Autodesk Fusion 360 part; units mm, degrees
(part 2 of 4)
  spline S375 degree 3 poles (7.1269, -2.7048) (6.3878, -3.105) (5.6098, -3.3959) (4.7931, -3.5774) knots 0 0 0 0 1 1 1 1
  spline S376 degree 3 poles (4.7931, -3.5774) (3.8693, -3.6414) (3.3958, -3.2084) (3.3726, -2.2787) knots 0 0 0 0 1 1 1 1
  spline S377 degree 3 poles (3.3726, -2.2787) (3.372, -1.9493) (3.4329, -1.6314) (3.5552, -1.3249) knots 0 0 0 0 1 1 1 1
  spline S378 degree 3 poles (3.5552, -1.3249) (3.871, -0.6919) (4.243, -0.0966) (4.6713, 0.4609) knots 0 0 0 0 1 1 1 1
  spline S379 degree 3 poles (4.6713, 0.4609) (4.606, 0.4941) (4.5384, 0.5211) (4.4684, 0.5421) knots 0 0 0 0 1 1 1 1
  spline S380 degree 3 poles (4.4684, 0.5421) (3.6102, -0.7693) (2.5279, -1.8584) (1.2215, -2.7251) knots 0 0 0 0 1 1 1 1
  spline S381 degree 3 poles (1.2215, -2.7251) (0.6448, -3.0748) (0.0225, -3.271) (-0.6454, -3.3136) knots 0 0 0 0 1 1 1 1
  spline S382 degree 3 poles (-0.6454, -3.3136) (-1.1329, -3.3261) (-1.4711, -3.1097) (-1.6601, -2.6642) knots 0 0 0 0 1 1 1 1
  spline S383 degree 3 poles (-1.6601, -2.6642) (-2.1725, -3.0359) (-2.7407, -3.2862) (-3.3647, -3.4151) knots 0 0 0 0 1 1 1 1
  spline S384 degree 3 poles (-3.3647, -3.4151) (-4.1602, -3.5477) (-4.8163, -3.3109) (-5.3331, -2.7048) knots 0 0 0 0 1 1 1 1
  spline S385 degree 3 poles (-5.3331, -2.7048) (-5.4007, -2.5695) (-5.4684, -2.4342) (-5.536, -2.299) knots 0 0 0 0 1 1 1 1
  spline S386 degree 3 poles (-5.536, -2.299) (-6.3793, -2.8663) (-7.2655, -3.3668) (-8.1944, -3.8006) knots 0 0 0 0 1 1 1 1
  spline S387 degree 3 poles (-8.1944, -3.8006) (-8.9496, -5.1315) (-9.8831, -6.3288) (-10.9948, -7.3925) knots 0 0 0 0 1 1 1 1
  spline S388 degree 3 poles (-10.9948, -7.3925) (-11.4326, -7.767) (-11.9332, -8.024) (-12.4965, -8.1636) knots 0 0 0 0 1 1 1 1
  spline S389 degree 3 poles (-12.4965, -8.1636) (-13.0579, -8.2343) (-13.4434, -8.0111) (-13.6532, -7.4939) knots 0 0 0 0 1 1 1 1
  spline S390 degree 3 poles (-13.6532, -7.4939) (-13.7714, -6.9994) (-13.7173, -6.5258) (-13.4908, -6.0734) knots 0 0 0 0 1 1 1 1
  spline S391 degree 3 poles (-13.4908, -6.0734) (-13.178, -5.5846) (-12.7924, -5.1584) (-12.3341, -4.795) knots 0 0 0 0 1 1 1 1
  spline S392 degree 3 poles (-12.3341, -4.795) (-11.6938, -4.29) (-11.0309, -3.8165) (-10.3454, -3.3745) knots 0 0 0 0 1 1 1 1
  spline S393 degree 3 poles (-10.3454, -3.3745) (-11.0952, -3.3991) (-11.6363, -3.0812) (-11.9689, -2.4207) knots 0 0 0 0 1 1 1 1
  spline S394 degree 3 poles (-11.9689, -2.4207) (-12.5057, -2.7974) (-13.0874, -3.0882) (-13.714, -3.2933) knots 0 0 0 0 1 1 1 1
  spline S395 degree 3 poles (-13.714, -3.2933) (-14.134, -3.37) (-14.5534, -3.37) (-14.9722, -3.2933) knots 0 0 0 0 1 1 1 1
  spline S396 degree 3 poles (-14.9722, -3.2933) (-15.2294, -3.1914) (-15.4458, -3.0358) (-15.6216, -2.8266) knots 0 0 0 0 1 1 1 1
  spline S397 degree 3 poles (-15.6216, -2.8266) (-16.2636, -3.2954) (-16.9806, -3.5051) (-17.7726, -3.4556) knots 0 0 0 0 1 1 1 1
  spline S398 degree 3 poles (-17.7726, -3.4556) (-18.8257, -3.1842) (-19.3196, -2.501) (-19.254, -1.4061) knots 0 0 0 0 1 1 1 1
  spline S399 degree 3 poles (-19.254, -1.4061) (-20.4254, -3.0432) (-22.0015, -3.6587) (-23.9822, -3.2527) knots 0 0 0 0 1 1 1 1
  spline S400 degree 3 poles (-23.9822, -3.2527) (-25.2943, -2.7924) (-25.9098, -1.8656) (-25.8289, -0.4726) knots 0 0 0 0 1 1 1 1
  spline S401 degree 3 poles (-25.8289, -0.4726) (-26.3281, -1.486) (-26.9843, -2.3856) (-27.7973, -3.1715) knots 0 0 0 0 1 1 1 1
  spline S402 degree 3 poles (-27.7973, -3.1715) (-28.5299, -3.7639) (-29.3551, -3.9533) (-30.273, -3.7397) knots 0 0 0 0 1 1 1 1
  spline S403 degree 3 poles (-30.273, -3.7397) (-30.803, -3.533) (-31.1886, -3.1745) (-31.4297, -2.6642) knots 0 0 0 0 1 1 1 1
  spline S404 degree 3 poles (-31.4297, -2.6642) (-31.4909, -2.3828) (-31.5044, -2.0987) (-31.4703, -1.8119) knots 0 0 0 0 1 1 1 1
  spline S405 degree 3 poles (-31.4703, -1.8119) (-31.2781, -1.361) (-30.9602, -1.246) (-30.5166, -1.4669) knots 0 0 0 0 1 1 1 1
  spline S406 degree 3 poles (-30.5166, -1.4669) (-30.4692, -1.5143) (-30.4219, -1.5616) (-30.3745, -1.609) knots 0 0 0 0 1 1 1 1
  spline S407 degree 3 poles (-30.3745, -1.609) (-30.3009, -1.7897) (-30.2197, -1.9656) (-30.131, -2.1366) knots 0 0 0 0 1 1 1 1
  spline S408 degree 3 poles (-30.131, -2.1366) (-29.5892, -2.3943) (-29.0819, -2.3335) (-28.609, -1.954) knots 0 0 0 0 1 1 1 1
  spline S409 degree 3 poles (-28.609, -1.954) (-28.0451, -1.3869) (-27.5648, -0.7579) (-27.1682, -0.0667) knots 0 0 0 0 1 1 1 1
  spline S410 degree 3 poles (-27.1682, -0.0667) (-26.4362, 1.3739) (-25.6313, 2.7674) (-24.7534, 4.1136) knots 0 0 0 0 1 1 1 1
  spline S411 degree 3 poles (-24.7534, 4.1136) (-25.9222, 4.7434) (-26.3213, 5.704) (-25.9507, 6.9952) knots 0 0 0 0 1 1 1 1
  spline S412 degree 3 poles (-25.9507, 6.9952) (-25.459, 8.0956) (-24.6134, 8.7111) (-23.414, 8.8418) knots 0 0 0 0 1 1 1 1
  spline S413 degree 3 poles (-23.414, 8.8418) (-22.6035, 8.8984) (-21.8189, 8.7834) (-21.0601, 8.4969) knots 0 0 0 0 1 1 1 1
  spline S414 degree 3 poles (-21.0601, 8.4969) (-20.2808, 9.0289) (-19.4285, 9.3671) (-18.5032, 9.5115) knots 0 0 0 0 1 1 1 1
  spline S415 degree 3 poles (-23.1299, 7.1575) (-23.7547, 7.0989) (-24.2485, 6.8148) (-24.6113, 6.3052) knots 0 0 0 0 1 1 1 1
  spline S416 degree 3 poles (-24.6113, 6.3052) (-24.6371, 6.2186) (-24.6235, 6.1374) (-24.5707, 6.0617) knots 0 0 0 0 1 1 1 1
  spline S417 degree 3 poles (-24.5707, 6.0617) (-24.4029, 5.8532) (-24.1932, 5.7247) (-23.9417, 5.6762) knots 0 0 0 0 1 1 1 1
  spline S418 degree 3 poles (-23.9417, 5.6762) (-23.5939, 6.1864) (-23.2151, 6.6734) (-22.8053, 7.1372) knots 0 0 0 0 1 1 1 1
  spline S419 degree 3 poles (-22.8053, 7.1372) (-22.9127, 7.1574) (-23.0209, 7.1642) (-23.1299, 7.1575) knots 0 0 0 0 1 1 1 1
  spline S420 degree 3 poles (-19.7207, 5.5341) (-19.7709, 5.4204) (-19.8317, 5.3122) (-19.9034, 5.2094) knots 0 0 0 0 1 1 1 1
  spline S421 degree 3 poles (-19.9034, 5.2094) (-20.3499, 4.7732) (-20.8437, 4.4012) (-21.3848, 4.0933) knots 0 0 0 0 1 1 1 1
  spline S422 degree 3 poles (-21.3848, 4.0933) (-21.9574, 3.7979) (-22.5662, 3.6356) (-23.2111, 3.6063) knots 0 0 0 0 1 1 1 1
  spline S423 degree 3 poles (-23.2111, 3.6063) (-23.6736, 2.9136) (-24.12, 2.2102) (-24.5504, 1.4958) knots 0 0 0 0 1 1 1 1
  spline S424 degree 3 poles (-24.5504, 1.4958) (-23.8967, 1.5933) (-23.2474, 1.5527) (-22.6023, 1.3741) knots 0 0 0 0 1 1 1 1
  spline S425 degree 3 poles (-22.6023, 1.3741) (-21.7597, 1.1706) (-21.4688, 0.6498) (-21.7297, -0.1885) knots 0 0 0 0 1 1 1 1
  spline S426 degree 3 poles (-21.7297, -0.1885) (-21.8822, -0.4816) (-22.1257, -0.6439) (-22.4603, -0.6755) knots 0 0 0 0 1 1 1 1
  spline S427 degree 3 poles (-22.4603, -0.6755) (-22.7996, -0.5567) (-23.1446, -0.4552) (-23.4952, -0.3711) knots 0 0 0 0 1 1 1 1
  spline S428 degree 3 poles (-23.4952, -0.3711) (-23.6981, -0.3441) (-23.9011, -0.3441) (-24.104, -0.3711) knots 0 0 0 0 1 1 1 1
  spline S429 degree 3 poles (-24.104, -0.3711) (-24.2834, -0.4288) (-24.3916, -0.5506) (-24.4287, -0.7364) knots 0 0 0 0 1 1 1 1
  spline S430 degree 3 poles (-24.4287, -0.7364) (-24.3891, -0.9653) (-24.2809, -1.1547) (-24.104, -1.3046) knots 0 0 0 0 1 1 1 1
  spline S431 degree 3 poles (-24.104, -1.3046) (-23.5604, -1.6749) (-22.9651, -1.7831) (-22.3182, -1.6293) knots 0 0 0 0 1 1 1 1
  spline S432 degree 3 poles (-22.3182, -1.6293) (-21.5751, -1.43) (-20.9595, -1.0309) (-20.4716, -0.432) knots 0 0 0 0 1 1 1 1
  spline S433 degree 3 poles (-20.4716, -0.432) (-19.3498, 1.1058) (-18.9575, 2.8104) (-19.2946, 4.6818) knots 0 0 0 0 1 1 1 1
  spline S434 degree 3 poles (-19.2946, 4.6818) (-19.3737, 5.0024) (-19.5157, 5.2865) (-19.7207, 5.5341) knots 0 0 0 0 1 1 1 1
  spline S435 degree 3 poles (3.1696, 1.6785) (2.4119, 0.9411) (1.634, 0.2241) (0.836, -0.4726) knots 0 0 0 0 1 1 1 1
  spline S436 degree 3 poles (0.836, -0.4726) (0.6736, -0.7161) (0.5113, -0.9596) (0.3489, -1.2031) knots 0 0 0 0 1 1 1 1
  spline S437 degree 3 poles (0.3489, -1.2031) (0.3091, -1.2542) (0.2956, -1.3083) (0.3083, -1.3655) knots 0 0 0 0 1 1 1 1
  spline S438 degree 3 poles (0.3083, -1.3655) (1.4523, -0.6846) (2.3993, 0.2083) (3.1493, 1.3132) knots 0 0 0 0 1 1 1 1
  spline S439 degree 3 poles (3.1493, 1.3132) (3.2168, 1.4374) (3.2236, 1.5591) (3.1696, 1.6785) knots 0 0 0 0 1 1 1 1
  spline S440 degree 3 poles (10.7999, 0.8667) (10.5828, 0.7924) (10.3665, 0.7045) (10.1506, 0.6029) knots 0 0 0 0 1 1 1 1
  spline S441 degree 3 poles (10.1506, 0.6029) (10.5418, 0.5621) (10.9071, 0.6432) (11.2464, 0.8464) knots 0 0 0 0 1 1 1 1
  spline S442 degree 3 poles (11.2464, 0.8464) (11.0982, 0.8667) (10.9493, 0.8734) (10.7999, 0.8667) knots 0 0 0 0 1 1 1 1
  spline S443 degree 3 poles (-1.1325, 0.6232) (-2.2555, 0.3285) (-3.2092, -0.2533) (-3.9938, -1.122) knots 0 0 0 0 1 1 1 1
  spline S444 degree 3 poles (-3.9938, -1.122) (-4.1157, -1.269) (-4.1969, -1.4313) (-4.2373, -1.609) knots 0 0 0 0 1 1 1 1
  spline S445 degree 3 poles (-4.2373, -1.609) (-4.1708, -1.7027) (-4.0829, -1.7636) (-3.9735, -1.7916) knots 0 0 0 0 1 1 1 1
  spline S446 degree 3 poles (-3.9735, -1.7916) (-3.69, -1.836) (-3.4194, -1.7954) (-3.1617, -1.6699) knots 0 0 0 0 1 1 1 1
  spline S447 degree 3 poles (-3.1617, -1.6699) (-2.1944, -1.1222) (-1.3624, -0.4119) (-0.6657, 0.4609) knots 0 0 0 0 1 1 1 1
  spline S448 degree 3 poles (-0.6657, 0.4609) (-0.6205, 0.512) (-0.6138, 0.5594) (-0.6454, 0.6029) knots 0 0 0 0 1 1 1 1
  spline S449 degree 3 poles (-0.6454, 0.6029) (-0.8072, 0.6232) (-0.9695, 0.63) (-1.1325, 0.6232) knots 0 0 0 0 1 1 1 1
  spline S450 degree 3 poles (-14.8099, 0.5826) (-16.001, 0.2541) (-16.9818, -0.3953) (-17.7523, -1.3655) knots 0 0 0 0 1 1 1 1
  spline S451 degree 3 poles (-17.7523, -1.3655) (-17.916, -1.5781) (-17.8686, -1.7202) (-17.6103, -1.7916) knots 0 0 0 0 1 1 1 1
  spline S452 degree 3 poles (-17.6103, -1.7916) (-17.4615, -1.8187) (-17.3127, -1.8187) (-17.1638, -1.7916) knots 0 0 0 0 1 1 1 1
  spline S453 degree 3 poles (-17.1638, -1.7916) (-16.7697, -1.6554) (-16.4044, -1.4661) (-16.068, -1.2234) knots 0 0 0 0 1 1 1 1
  spline S454 degree 3 poles (-16.068, -1.2234) (-15.3561, -0.7146) (-14.7067, -0.1328) (-14.1199, 0.5218) knots 0 0 0 0 1 1 1 1
  spline S455 degree 3 poles (-14.1199, 0.5218) (-14.3424, 0.5806) (-14.5724, 0.6009) (-14.8099, 0.5826) knots 0 0 0 0 1 1 1 1
  spline S456 degree 3 poles (16.8878, 0.5826) (16.6881, 0.5291) (16.4852, 0.4682) (16.279, 0.4) knots 0 0 0 0 1 1 1 1
  spline S457 degree 3 poles (16.279, 0.4) (15.2944, -0.0031) (14.4896, -0.6321) (13.8642, -1.4872) knots 0 0 0 0 1 1 1 1
  spline S458 degree 3 poles (13.8642, -1.4872) (13.8341, -1.566) (13.8406, -1.6404) (13.8844, -1.7105) knots 0 0 0 0 1 1 1 1
  spline S459 degree 3 poles (13.8844, -1.7105) (14.1799, -1.8416) (14.4774, -1.8416) (14.7773, -1.7105) knots 0 0 0 0 1 1 1 1
  spline S460 degree 3 poles (14.7773, -1.7105) (15.1357, -1.5382) (15.4738, -1.3352) (15.792, -1.1017) knots 0 0 0 0 1 1 1 1
  spline S461 degree 3 poles (15.792, -1.1017) (16.4174, -0.6385) (16.9925, -0.1177) (17.5169, 0.4609) knots 0 0 0 0 1 1 1 1
  spline S462 degree 3 poles (17.5169, 0.4609) (17.5364, 0.4994) (17.5433, 0.5399) (17.5372, 0.5826) knots 0 0 0 0 1 1 1 1
  spline S463 degree 3 poles (17.5372, 0.5826) (17.3208, 0.5826) (17.1041, 0.5826) (16.8878, 0.5826) knots 0 0 0 0 1 1 1 1
  spline S464 degree 3 poles (11.0029, -1.2031) (10.1522, -1.325) (9.3271, -1.2303) (8.5271, -0.919) knots 0 0 0 0 1 1 1 1
  spline S465 degree 3 poles (8.5271, -0.919) (8.4602, -0.9709) (8.4127, -1.0386) (8.3851, -1.122) knots 0 0 0 0 1 1 1 1
  spline S466 degree 3 poles (8.3851, -1.122) (8.3376, -1.264) (8.2901, -1.4061) (8.243, -1.5481) knots 0 0 0 0 1 1 1 1
  spline S467 degree 3 poles (8.243, -1.5481) (8.2532, -1.5993) (8.2804, -1.6399) (8.3242, -1.6699) knots 0 0 0 0 1 1 1 1
  spline S468 degree 3 poles (8.3242, -1.6699) (9.2719, -1.8362) (10.1648, -1.6806) (11.0029, -1.2031) knots 0 0 0 0 1 1 1 1
  spline S469 degree 3 poles (-18.5032, 9.3492) (-17.6562, 9.4316) (-16.858, 9.276) (-16.1086, 8.8824) knots 0 0 0 0 1 1 1 1
  spline S470 degree 3 poles (-16.1086, 8.8824) (-15.7821, 8.6642) (-15.5454, 8.3733) (-15.3984, 8.0098) knots 0 0 0 0 1 1 1 1
  spline S471 degree 3 poles (-15.3984, 8.0098) (-15.3446, 7.5901) (-15.5273, 7.394) (-15.9463, 7.4213) knots 0 0 0 0 1 1 1 1
  spline S472 degree 3 poles (-15.9463, 7.4213) (-16.0104, 7.45) (-16.0713, 7.4838) (-16.1289, 7.5228) knots 0 0 0 0 1 1 1 1
  spline S473 degree 3 poles (-16.1289, 7.5228) (-16.3363, 8.0225) (-16.7083, 8.3133) (-17.245, 8.3954) knots 0 0 0 0 1 1 1 1
  spline S474 degree 3 poles (-17.245, 8.3954) (-18.2437, 8.5762) (-19.1772, 8.4071) (-20.0454, 7.8881) knots 0 0 0 0 1 1 1 1
  spline S475 degree 3 poles (-20.0454, 7.8881) (-18.6024, 6.8964) (-17.8854, 5.5164) (-17.8944, 3.7483) knots 0 0 0 0 1 1 1 1
  spline S476 degree 3 poles (-17.8944, 3.7483) (-17.9234, 1.9636) (-18.4442, 0.3401) (-19.4569, -1.122) knots 0 0 0 0 1 1 1 1
  spline S477 degree 3 poles (-19.4569, -1.122) (-20.0686, -1.91) (-20.8465, -2.4579) (-21.7906, -2.7657) knots 0 0 0 0 1 1 1 1
  spline S478 degree 3 poles (-21.7906, -2.7657) (-22.926, -3.1064) (-23.9677, -2.9305) (-24.9157, -2.2381) knots 0 0 0 0 1 1 1 1
  spline S479 degree 3 poles (-24.9157, -2.2381) (-25.5232, -1.656) (-25.7599, -0.9457) (-25.626, -0.1073) knots 0 0 0 0 1 1 1 1
  spline S480 degree 3 poles (-25.626, -0.1073) (-25.4125, 0.6474) (-24.9186, 1.087) (-24.1446, 1.2117) knots 0 0 0 0 1 1 1 1
  spline S481 degree 3 poles (-24.1446, 1.2117) (-23.6207, 1.2236) (-23.1066, 1.156) (-22.6023, 1.0088) knots 0 0 0 0 1 1 1 1
  spline S482 degree 3 poles (-22.6023, 1.0088) (-22.3358, 0.9581) (-22.1397, 0.816) (-22.0138, 0.5826) knots 0 0 0 0 1 1 1 1
  spline S483 degree 3 poles (-22.0138, 0.5826) (-21.9865, 0.1636) (-22.1826, -0.019) (-22.6023, 0.0347) knots 0 0 0 0 1 1 1 1
  spline S484 degree 3 poles (-22.6023, 0.0347) (-23.1335, 0.2942) (-23.6882, 0.3754) (-24.2664, 0.2782) knots 0 0 0 0 1 1 1 1
  spline S485 degree 3 poles (-24.2664, 0.2782) (-24.6176, 0.1035) (-24.7799, -0.1806) (-24.7534, -0.5741) knots 0 0 0 0 1 1 1 1
  spline S486 degree 3 poles (-24.7534, -0.5741) (-24.7601, -1.0409) (-24.5707, -1.4061) (-24.1852, -1.6699) knots 0 0 0 0 1 1 1 1
  spline S487 degree 3 poles (-24.1852, -1.6699) (-23.6603, -1.9874) (-23.0921, -2.0957) (-22.4806, -1.9946) knots 0 0 0 0 1 1 1 1
  spline S488 degree 3 poles (-22.4806, -1.9946) (-21.5608, -1.8425) (-20.81, -1.4028) (-20.2281, -0.6755) knots 0 0 0 0 1 1 1 1
  spline S489 degree 3 poles (-20.2281, -0.6755) (-19.4037, 0.4439) (-18.9302, 1.702) (-18.8076, 3.099) knots 0 0 0 0 1 1 1 1
  spline S490 degree 3 poles (-18.8076, 3.099) (-18.6631, 4.1951) (-18.8796, 5.2098) (-19.4569, 6.1429) knots 0 0 0 0 1 1 1 1
  spline S491 degree 3 poles (-19.4569, 6.1429) (-19.8338, 6.6553) (-20.3072, 7.0476) (-20.8774, 7.3199) knots 0 0 0 0 1 1 1 1
  spline S492 degree 3 poles (-20.8774, 7.3199) (-21.5825, 6.7128) (-22.198, 6.0296) (-22.7241, 5.2703) knots 0 0 0 0 1 1 1 1
  spline S493 degree 3 poles (-22.7241, 5.2703) (-22.397, 5.3207) (-22.0859, 5.429) (-21.7906, 5.595) knots 0 0 0 0 1 1 1 1
  spline S494 degree 3 poles (-21.7906, 5.595) (-21.4151, 5.8621) (-21.0633, 6.1598) (-20.7354, 6.4879) knots 0 0 0 0 1 1 1 1
  spline S495 degree 3 poles (-20.7354, 6.4879) (-20.4696, 6.6428) (-20.2464, 6.5955) (-20.0657, 6.3458) knots 0 0 0 0 1 1 1 1
  spline S496 degree 3 poles (-20.0657, 6.3458) (-20.0235, 6.1453) (-20.0505, 5.9559) (-20.1469, 5.7776) knots 0 0 0 0 1 1 1 1
  spline S497 degree 3 poles (-20.1469, 5.7776) (-21.0651, 4.845) (-22.1745, 4.3174) (-23.4749, 4.1948) knots 0 0 0 0 1 1 1 1
  spline S498 degree 3 poles (-23.4749, 4.1948) (-23.8673, 3.5725) (-24.2596, 2.9501) (-24.6519, 2.3278) knots 0 0 0 0 1 1 1 1
  spline S499 degree 3 poles (-24.6519, 2.3278) (-25.318, 1.1172) (-25.9945, -0.0868) (-26.6812, -1.2843) knots 0 0 0 0 1 1 1 1
  spline S500 degree 3 poles (-26.6812, -1.2843) (-26.996, -1.7575) (-27.3545, -2.1972) (-27.7567, -2.6033) knots 0 0 0 0 1 1 1 1
  spline S501 degree 3 poles (-27.7567, -2.6033) (-28.3894, -3.1795) (-29.1335, -3.423) (-29.9889, -3.3339) knots 0 0 0 0 1 1 1 1
  spline S502 degree 3 poles (-29.9889, -3.3339) (-30.5331, -3.1815) (-30.9457, -2.8636) (-31.2268, -2.3801) knots 0 0 0 0 1 1 1 1
  spline S503 degree 3 poles (-31.2268, -2.3801) (-31.3301, -2.1673) (-31.3437, -1.9508) (-31.2674, -1.7308) knots 0 0 0 0 1 1 1 1
  spline S504 degree 3 poles (-31.2674, -1.7308) (-31.061, -1.5028) (-30.8243, -1.469) (-30.5571, -1.6293) knots 0 0 0 0 1 1 1 1
  spline S505 degree 3 poles (-30.5571, -1.6293) (-30.4671, -1.791) (-30.3927, -1.9601) (-30.3339, -2.1366) knots 0 0 0 0 1 1 1 1
  spline S506 degree 3 poles (-30.3339, -2.1366) (-30.0544, -2.4455) (-29.7094, -2.547) (-29.299, -2.441) knots 0 0 0 0 1 1 1 1
  spline S507 degree 3 poles (-29.299, -2.441) (-28.8702, -2.3503) (-28.5117, -2.1406) (-28.2235, -1.8119) knots 0 0 0 0 1 1 1 1
  spline S508 degree 3 poles (-28.2235, -1.8119) (-27.8963, -1.4415) (-27.5986, -1.0491) (-27.3306, -0.6349) knots 0 0 0 0 1 1 1 1
  spline S509 degree 3 poles (-27.3306, -0.6349) (-26.7386, 0.4002) (-26.1568, 1.4419) (-25.5854, 2.4902) knots 0 0 0 0 1 1 1 1
  spline S510 degree 3 poles (-25.5854, 2.4902) (-25.1829, 3.1464) (-24.7703, 3.7958) (-24.3475, 4.4383) knots 0 0 0 0 1 1 1 1
  spline S511 degree 3 poles (-24.3475, 4.4383) (-25.5575, 4.8706) (-26.0378, 5.7093) (-25.7883, 6.9546) knots 0 0 0 0 1 1 1 1
  spline S512 degree 3 poles (-25.7883, 6.9546) (-25.3369, 7.9894) (-24.5455, 8.5644) (-23.414, 8.6795) knots 0 0 0 0 1 1 1 1
  spline S513 degree 3 poles (-23.414, 8.6795) (-22.5987, 8.7342) (-21.8073, 8.6191) (-21.0398, 8.3345) knots 0 0 0 0 1 1 1 1
  spline S514 degree 3 poles (-21.0398, 8.3345) (-20.261, 8.8494) (-19.4155, 9.1876) (-18.5032, 9.3492) knots 0 0 0 0 1 1 1 1
  spline S515 degree 3 poles (-23.1299, 7.1575) (-23.7547, 7.0989) (-24.2485, 6.8148) (-24.6113, 6.3052) knots 0 0 0 0 1 1 1 1
  spline S516 degree 3 poles (-24.6113, 6.3052) (-24.6371, 6.2186) (-24.6235, 6.1374) (-24.5707, 6.0617) knots 0 0 0 0 1 1 1 1
  spline S517 degree 3 poles (-24.5707, 6.0617) (-24.4029, 5.8532) (-24.1932, 5.7247) (-23.9417, 5.6762) knots 0 0 0 0 1 1 1 1
  spline S518 degree 3 poles (-23.9417, 5.6762) (-23.5939, 6.1864) (-23.2151, 6.6734) (-22.8053, 7.1372) knots 0 0 0 0 1 1 1 1
  spline S519 degree 3 poles (-22.8053, 7.1372) (-22.9127, 7.1574) (-23.0209, 7.1642) (-23.1299, 7.1575) knots 0 0 0 0 1 1 1 1
  spline S520 degree 3 poles (-23.3735, 7.8069) (-23.1026, 7.8136) (-22.832, 7.8069) (-22.5617, 7.7866) knots 0 0 0 0 1 1 1 1
  spline S521 degree 3 poles (-22.5617, 7.7866) (-22.3197, 7.7733) (-22.0897, 7.7192) (-21.8718, 7.6243) knots 0 0 0 0 1 1 1 1
  spline S522 degree 3 poles (-21.8718, 7.6243) (-22.5639, 6.9085) (-23.193, 6.1441) (-23.759, 5.3312) knots 0 0 0 0 1 1 1 1
  spline S523 degree 3 poles (-23.759, 5.3312) (-23.789, 5.2876) (-23.8296, 5.2605) (-23.8808, 5.25) knots 0 0 0 0 1 1 1 1
  spline S524 degree 3 poles (-23.8808, 5.25) (-24.3842, 5.3593) (-24.7495, 5.6434) (-24.9766, 6.1023) knots 0 0 0 0 1 1 1 1
  spline S525 degree 3 poles (-24.9766, 6.1023) (-25.0395, 6.4115) (-24.9854, 6.6956) (-24.8143, 6.9546) knots 0 0 0 0 1 1 1 1
  spline S526 degree 3 poles (-24.8143, 6.9546) (-24.4328, 7.4123) (-23.9525, 7.6964) (-23.3735, 7.8069) knots 0 0 0 0 1 1 1 1
  spline S527 degree 3 poles (-23.1299, 7.1575) (-23.7547, 7.0989) (-24.2485, 6.8148) (-24.6113, 6.3052) knots 0 0 0 0 1 1 1 1
  spline S528 degree 3 poles (-24.6113, 6.3052) (-24.6371, 6.2186) (-24.6235, 6.1374) (-24.5707, 6.0617) knots 0 0 0 0 1 1 1 1
  spline S529 degree 3 poles (-24.5707, 6.0617) (-24.4029, 5.8532) (-24.1932, 5.7247) (-23.9417, 5.6762) knots 0 0 0 0 1 1 1 1
  spline S530 degree 3 poles (-23.9417, 5.6762) (-23.5939, 6.1864) (-23.2151, 6.6734) (-22.8053, 7.1372) knots 0 0 0 0 1 1 1 1
  spline S531 degree 3 poles (-22.8053, 7.1372) (-22.9127, 7.1574) (-23.0209, 7.1642) (-23.1299, 7.1575) knots 0 0 0 0 1 1 1 1
  spline S532 degree 3 poles (-23.3735, 7.3199) (-23.0594, 7.3343) (-22.7482, 7.314) (-22.44, 7.259) knots 0 0 0 0 1 1 1 1
  spline S533 degree 3 poles (-22.44, 7.259) (-22.9598, 6.6988) (-23.4333, 6.1036) (-23.8605, 5.4732) knots 0 0 0 0 1 1 1 1
  spline S534 degree 3 poles (-23.8605, 5.4732) (-24.2998, 5.5197) (-24.6177, 5.743) (-24.8143, 6.1429) knots 0 0 0 0 1 1 1 1
  spline S535 degree 3 poles (-24.8143, 6.1429) (-24.7735, 6.4332) (-24.6314, 6.67) (-24.3881, 6.8531) knots 0 0 0 0 1 1 1 1
  spline S536 degree 3 poles (-24.3881, 6.8531) (-24.0772, 7.0759) (-23.739, 7.2315) (-23.3735, 7.3199) knots 0 0 0 0 1 1 1 1
  spline S537 degree 3 poles (-23.1299, 7.1575) (-23.7547, 7.0989) (-24.2485, 6.8148) (-24.6113, 6.3052) knots 0 0 0 0 1 1 1 1
  spline S538 degree 3 poles (-24.6113, 6.3052) (-24.6371, 6.2186) (-24.6235, 6.1374) (-24.5707, 6.0617) knots 0 0 0 0 1 1 1 1
  spline S539 degree 3 poles (-24.5707, 6.0617) (-24.4029, 5.8532) (-24.1932, 5.7247) (-23.9417, 5.6762) knots 0 0 0 0 1 1 1 1
  spline S540 degree 3 poles (-23.9417, 5.6762) (-23.5939, 6.1864) (-23.2151, 6.6734) (-22.8053, 7.1372) knots 0 0 0 0 1 1 1 1
  spline S541 degree 3 poles (-22.8053, 7.1372) (-22.9127, 7.1574) (-23.0209, 7.1642) (-23.1299, 7.1575) knots 0 0 0 0 1 1 1 1
  spline S542 degree 3 poles (-20.8977, 6.7923) (-20.8197, 6.7803) (-20.752, 6.7465) (-20.6948, 6.6908) knots 0 0 0 0 1 1 1 1
  spline S543 degree 3 poles (-20.6948, 6.6908) (-21.0044, 6.4489) (-21.302, 6.1919) (-21.5877, 5.9197) knots 0 0 0 0 1 1 1 1
  spline S544 degree 3 poles (-21.5877, 5.9197) (-21.6905, 5.8412) (-21.7988, 5.787) (-21.9124, 5.7573) knots 0 0 0 0 1 1 1 1
  spline S545 degree 3 poles (-21.9124, 5.7573) (-21.5931, 6.1239) (-21.2549, 6.4689) (-20.8977, 6.7923) knots 0 0 0 0 1 1 1 1
  spline S546 degree 3 poles (-19.8831, 6.0211) (-19.567, 5.7152) (-19.3302, 5.3499) (-19.1728, 4.9253) knots 0 0 0 0 1 1 1 1
  spline S547 degree 3 poles (-19.1728, 4.9253) (-18.7456, 2.9677) (-19.1109, 1.1684) (-20.2687, -0.4726) knots 0 0 0 0 1 1 1 1
  spline S548 degree 3 poles (-20.2687, -0.4726) (-21.0585, -1.5163) (-22.107, -1.9695) (-23.414, -1.8322) knots 0 0 0 0 1 1 1 1
  spline S549 degree 3 poles (-23.414, -1.8322) (-23.8998, -1.7247) (-24.2718, -1.4609) (-24.5302, -1.0408) knots 0 0 0 0 1 1 1 1
  spline S550 degree 3 poles (-24.5302, -1.0408) (-24.6707, -0.4829) (-24.4542, -0.1853) (-23.8808, -0.1479) knots 0 0 0 0 1 1 1 1
  spline S551 degree 3 poles (-23.8808, -0.1479) (-23.4481, -0.1698) (-23.0355, -0.2713) (-22.6429, -0.4523) knots 0 0 0 0 1 1 1 1
  spline S552 degree 3 poles (-22.6429, -0.4523) (-22.1845, -0.5147) (-21.9139, -0.3185) (-21.8312, 0.1362) knots 0 0 0 0 1 1 1 1
  spline S553 degree 3 poles (-21.8312, 0.1362) (-21.758, 0.5319) (-21.8933, 0.8363) (-22.2371, 1.0494) knots 0 0 0 0 1 1 1 1
  spline S554 degree 3 poles (-22.2371, 1.0494) (-22.9866, 1.3584) (-23.7578, 1.4395) (-24.5504, 1.2929) knots 0 0 0 0 1 1 1 1
  spline S555 degree 3 poles (-24.5504, 1.2929) (-24.6825, 1.2512) (-24.8043, 1.1903) (-24.9157, 1.1103) knots 0 0 0 0 1 1 1 1
  spline S556 degree 3 poles (-24.9157, 1.1103) (-24.9572, 1.1306) (-24.9639, 1.1577) (-24.936, 1.1914) knots 0 0 0 0 1 1 1 1
  spline S557 degree 3 poles (-24.936, 1.1914) (-24.4258, 2.0734) (-23.8914, 2.9392) (-23.3329, 3.7889) knots 0 0 0 0 1 1 1 1
  spline S558 degree 3 poles (-23.3329, 3.7889) (-21.9954, 3.8793) (-20.8793, 4.4205) (-19.9846, 5.4123) knots 0 0 0 0 1 1 1 1
  spline S559 degree 3 poles (-19.9846, 5.4123) (-19.8975, 5.6055) (-19.8637, 5.8084) (-19.8831, 6.0211) knots 0 0 0 0 1 1 1 1
  spline S560 degree 3 poles (-19.7207, 5.5341) (-19.7709, 5.4204) (-19.8317, 5.3122) (-19.9034, 5.2094) knots 0 0 0 0 1 1 1 1
  spline S561 degree 3 poles (-19.9034, 5.2094) (-20.3499, 4.7732) (-20.8437, 4.4012) (-21.3848, 4.0933) knots 0 0 0 0 1 1 1 1
  spline S562 degree 3 poles (-21.3848, 4.0933) (-21.9574, 3.7979) (-22.5662, 3.6356) (-23.2111, 3.6063) knots 0 0 0 0 1 1 1 1
  spline S563 degree 3 poles (-23.2111, 3.6063) (-23.6736, 2.9136) (-24.12, 2.2102) (-24.5504, 1.4958) knots 0 0 0 0 1 1 1 1
  spline S564 degree 3 poles (-24.5504, 1.4958) (-23.8967, 1.5933) (-23.2474, 1.5527) (-22.6023, 1.3741) knots 0 0 0 0 1 1 1 1
  spline S565 degree 3 poles (-22.6023, 1.3741) (-21.7597, 1.1706) (-21.4688, 0.6498) (-21.7297, -0.1885) knots 0 0 0 0 1 1 1 1
  spline S566 degree 3 poles (-21.7297, -0.1885) (-21.8822, -0.4816) (-22.1257, -0.6439) (-22.4603, -0.6755) knots 0 0 0 0 1 1 1 1
  spline S567 degree 3 poles (-22.4603, -0.6755) (-22.7996, -0.5567) (-23.1446, -0.4552) (-23.4952, -0.3711) knots 0 0 0 0 1 1 1 1
  spline S568 degree 3 poles (-23.4952, -0.3711) (-23.6981, -0.3441) (-23.9011, -0.3441) (-24.104, -0.3711) knots 0 0 0 0 1 1 1 1
  spline S569 degree 3 poles (-24.104, -0.3711) (-24.2834, -0.4288) (-24.3916, -0.5506) (-24.4287, -0.7364) knots 0 0 0 0 1 1 1 1
  spline S570 degree 3 poles (-24.4287, -0.7364) (-24.3891, -0.9653) (-24.2809, -1.1547) (-24.104, -1.3046) knots 0 0 0 0 1 1 1 1
  spline S571 degree 3 poles (-24.104, -1.3046) (-23.5604, -1.6749) (-22.9651, -1.7831) (-22.3182, -1.6293) knots 0 0 0 0 1 1 1 1
  spline S572 degree 3 poles (-22.3182, -1.6293) (-21.5751, -1.43) (-20.9595, -1.0309) (-20.4716, -0.432) knots 0 0 0 0 1 1 1 1
  spline S573 degree 3 poles (-20.4716, -0.432) (-19.3498, 1.1058) (-18.9575, 2.8104) (-19.2946, 4.6818) knots 0 0 0 0 1 1 1 1
  spline S574 degree 3 poles (-19.2946, 4.6818) (-19.3737, 5.0024) (-19.5157, 5.2865) (-19.7207, 5.5341) knots 0 0 0 0 1 1 1 1
  spline S575 degree 3 poles (25.6543, 1.1914) (25.6413, 1.0535) (25.6547, 0.9182) (25.6949, 0.7856) knots 0 0 0 0 1 1 1 1
  spline S576 degree 3 poles (25.6949, 0.7856) (25.7197, 0.7906) (25.7331, 0.8041) (25.7355, 0.8262) knots 0 0 0 0 1 1 1 1
  spline S577 degree 3 poles (25.7355, 0.8262) (26.3008, 1.3291) (26.9502, 1.6876) (27.6836, 1.9017) knots 0 0 0 0 1 1 1 1
  spline S578 degree 3 poles (27.6836, 1.9017) (28.2465, 2.043) (28.7133, 1.9009) (29.0838, 1.4755) knots 0 0 0 0 1 1 1 1
  spline S579 degree 3 poles (29.0838, 1.4755) (29.111, 1.4214) (29.1378, 1.3673) (29.165, 1.3132) knots 0 0 0 0 1 1 1 1
  spline S580 degree 3 poles (29.165, 1.3132) (29.2364, 0.8962) (29.1686, 0.5039) (28.9621, 0.1362) knots 0 0 0 0 1 1 1 1
  spline S581 degree 3 poles (28.9621, 0.1362) (28.6325, -0.4008) (28.2538, -0.9013) (27.8257, -1.3655) knots 0 0 0 0 1 1 1 1
  spline S582 degree 3 poles (27.8257, -1.3655) (27.6808, -1.5471) (27.5793, -1.75) (27.5213, -1.9743) knots 0 0 0 0 1 1 1 1
  spline S583 degree 3 poles (27.5213, -1.9743) (28.0615, -1.9769) (28.5619, -1.8349) (29.0229, -1.5481) knots 0 0 0 0 1 1 1 1
  spline S584 degree 3 poles (29.0229, -1.5481) (29.5855, -1.1889) (30.1131, -0.783) (30.6058, -0.3305) knots 0 0 0 0 1 1 1 1
  spline S585 degree 3 poles (30.6058, -0.3305) (31.0843, -0.3189) (31.2397, -0.5421) (31.0725, -1.0002) knots 0 0 0 0 1 1 1 1
  spline S586 degree 3 poles (31.0725, -1.0002) (30.2673, -1.8528) (29.3001, -2.4412) (28.1706, -2.7657) knots 0 0 0 0 1 1 1 1
  spline S587 degree 3 poles (28.1706, -2.7657) (27.8865, -2.7928) (27.6024, -2.7928) (27.3183, -2.7657) knots 0 0 0 0 1 1 1 1
  spline S588 degree 3 poles (27.3183, -2.7657) (26.7538, -2.5485) (26.5712, -2.1494) (26.7704, -1.5684) knots 0 0 0 0 1 1 1 1
  spline S589 degree 3 poles (26.7704, -1.5684) (26.8715, -1.3388) (26.9932, -1.1224) (27.1357, -0.919) knots 0 0 0 0 1 1 1 1
  spline S590 degree 3 poles (27.1357, -0.919) (27.4912, -0.5366) (27.8159, -0.1307) (28.1098, 0.2985) knots 0 0 0 0 1 1 1 1
  spline S591 degree 3 poles (28.1098, 0.2985) (28.2104, 0.4664) (28.2916, 0.6422) (28.3533, 0.8262) knots 0 0 0 0 1 1 1 1
  spline S592 degree 3 poles (28.3533, 0.8262) (28.3841, 0.9182) (28.3772, 1.0062) (28.333, 1.09) knots 0 0 0 0 1 1 1 1
  spline S593 degree 3 poles (28.333, 1.09) (28.1434, 1.117) (27.9543, 1.117) (27.7648, 1.09) knots 0 0 0 0 1 1 1 1
  spline S594 degree 3 poles (27.7648, 1.09) (27.0821, 0.8262) (26.4733, 0.4474) (25.9384, -0.0464) knots 0 0 0 0 1 1 1 1
  spline S595 degree 3 poles (25.9384, -0.0464) (24.9822, -0.9481) (24.1165, -1.9222) (23.3409, -2.9686) knots 0 0 0 0 1 1 1 1
  spline S596 degree 3 poles (23.3409, -2.9686) (23.2687, -2.9668) (23.2009, -2.9398) (23.138, -2.8874) knots 0 0 0 0 1 1 1 1
  spline S597 degree 3 poles (23.138, -2.8874) (22.996, -2.7725) (22.8539, -2.6574) (22.7119, -2.5425) knots 0 0 0 0 1 1 1 1
  spline S598 degree 3 poles (22.7119, -2.5425) (22.6847, -2.5019) (22.6847, -2.4613) (22.7119, -2.4207) knots 0 0 0 0 1 1 1 1
  spline S599 degree 3 poles (22.7119, -2.4207) (23.1599, -1.9049) (23.593, -1.3773) (24.0106, -0.8379) knots 0 0 0 0 1 1 1 1
  spline S600 degree 3 poles (24.0106, -0.8379) (24.3779, -0.3606) (24.6482, 0.167) (24.8223, 0.745) knots 0 0 0 0 1 1 1 1
  spline S601 degree 3 poles (24.8223, 0.745) (24.8613, 0.9102) (24.841, 1.0658) (24.7614, 1.2117) knots 0 0 0 0 1 1 1 1
  spline S602 degree 3 poles (24.7614, 1.2117) (24.4481, 1.2484) (24.1506, 1.1943) (23.8685, 1.0494) knots 0 0 0 0 1 1 1 1
  spline S603 degree 3 poles (23.8685, 1.0494) (23.2687, 0.7596) (22.7005, 0.4214) (22.1639, 0.0347) knots 0 0 0 0 1 1 1 1
  spline S604 degree 3 poles (22.1639, 0.0347) (21.638, -0.3693) (21.1241, -0.7887) (20.6217, -1.2234) knots 0 0 0 0 1 1 1 1
  spline S605 degree 3 poles (20.6217, -1.2234) (20.0032, -1.8691) (19.3607, -2.4846) (18.6939, -3.0701) knots 0 0 0 0 1 1 1 1
  spline S606 degree 3 poles (18.6939, -3.0701) (18.5449, -2.9483) (18.3964, -2.8266) (18.2474, -2.7048) knots 0 0 0 0 1 1 1 1
  spline S607 degree 3 poles (18.2474, -2.7048) (17.7502, -2.8778) (17.2429, -2.9116) (16.7254, -2.8063) knots 0 0 0 0 1 1 1 1
  spline S608 degree 3 poles (16.7254, -2.8063) (16.4641, -2.6936) (16.2676, -2.5109) (16.137, -2.2584) knots 0 0 0 0 1 1 1 1
  spline S609 degree 3 poles (16.137, -2.2584) (15.5955, -2.6689) (14.9868, -2.9124) (14.3106, -2.9889) knots 0 0 0 0 1 1 1 1
  spline S610 degree 3 poles (14.3106, -2.9889) (13.3978, -2.9757) (12.8227, -2.5292) (12.5857, -1.6496) knots 0 0 0 0 1 1 1 1
  spline S611 degree 3 poles (12.5857, -1.6496) (11.7748, -2.1903) (10.8953, -2.5758) (9.9476, -2.8063) knots 0 0 0 0 1 1 1 1
  spline S612 degree 3 poles (9.9476, -2.8063) (9.2974, -2.9375) (8.6477, -2.9375) (7.9995, -2.8063) knots 0 0 0 0 1 1 1 1
  spline S613 degree 3 poles (7.9995, -2.8063) (7.648, -2.6849) (7.3842, -2.4617) (7.2081, -2.1366) knots 0 0 0 0 1 1 1 1
  spline S614 degree 3 poles (7.2081, -2.1366) (6.454, -2.5847) (5.6489, -2.9027) (4.7931, -3.0904) knots 0 0 0 0 1 1 1 1
  spline S615 degree 3 poles (4.7931, -3.0904) (4.0331, -3.1844) (3.6137, -2.8529) (3.5349, -2.096) knots 0 0 0 0 1 1 1 1
  spline S616 degree 3 poles (3.5349, -2.096) (3.5916, -1.662) (3.7337, -1.2562) (3.9611, -0.8785) knots 0 0 0 0 1 1 1 1
  spline S617 degree 3 poles (3.9611, -0.8785) (4.3387, -0.2651) (4.7513, 0.3234) (5.1989, 0.887) knots 0 0 0 0 1 1 1 1
  spline S618 degree 3 poles (5.1989, 0.887) (4.9418, 0.9344) (4.6848, 0.9818) (4.4278, 1.0291) knots 0 0 0 0 1 1 1 1
  spline S619 degree 3 poles (4.4278, 1.0291) (4.2269, 0.8067) (4.0443, 0.5632) (3.8799, 0.2985) knots 0 0 0 0 1 1 1 1
  spline S620 degree 3 poles (3.8799, 0.2985) (3.6364, 0.0009) (3.3929, -0.2967) (3.1493, -0.5943) knots 0 0 0 0 1 1 1 1
  spline S621 degree 3 poles (3.1493, -0.5943) (2.557, -1.2244) (1.9008, -1.7723) (1.1809, -2.2381) knots 0 0 0 0 1 1 1 1
  spline S622 degree 3 poles (1.1809, -2.2381) (0.8389, -2.4226) (0.4872, -2.585) (0.1257, -2.7251) knots 0 0 0 0 1 1 1 1
  spline S623 degree 3 poles (0.1257, -2.7251) (-0.2786, -2.8306) (-0.6845, -2.8441) (-1.0919, -2.7657) knots 0 0 0 0 1 1 1 1
  spline S624 degree 3 poles (-1.0919, -2.7657) (-1.3711, -2.5944) (-1.5132, -2.3441) (-1.518, -2.0149) knots 0 0 0 0 1 1 1 1
  spline S625 degree 3 poles (-1.518, -2.0149) (-2.282, -2.716) (-3.1816, -3.0204) (-4.217, -2.928) knots 0 0 0 0 1 1 1 1
  spline S626 degree 3 poles (-4.217, -2.928) (-4.858, -2.7604) (-5.2707, -2.3613) (-5.4548, -1.7308) knots 0 0 0 0 1 1 1 1
  spline S627 degree 3 poles (-5.4548, -1.7308) (-6.3534, -2.3301) (-7.2936, -2.8645) (-8.2756, -3.3339) knots 0 0 0 0 1 1 1 1
  spline S628 degree 3 poles (-8.2756, -3.3339) (-9.013, -4.613) (-9.9058, -5.7764) (-10.9542, -6.8243) knots 0 0 0 0 1 1 1 1
  spline S629 degree 3 poles (-10.9542, -6.8243) (-11.3533, -7.1958) (-11.8133, -7.4664) (-12.3341, -7.636) knots 0 0 0 0 1 1 1 1
  spline S630 degree 3 poles (-12.3341, -7.636) (-13.1638, -7.7801) (-13.5629, -7.4351) (-13.5314, -6.601) knots 0 0 0 0 1 1 1 1
  spline S631 degree 3 poles (-13.5314, -6.601) (-13.4524, -6.3349) (-13.3307, -6.0914) (-13.1661, -5.8705) knots 0 0 0 0 1 1 1 1
  spline S632 degree 3 poles (-13.1661, -5.8705) (-12.8347, -5.4849) (-12.4762, -5.1264) (-12.0906, -4.795) knots 0 0 0 0 1 1 1 1
  spline S633 degree 3 poles (-12.0906, -4.795) (-11.1036, -4.0387) (-10.0619, -3.3622) (-8.9655, -2.7657) knots 0 0 0 0 1 1 1 1
  spline S634 degree 3 poles (-8.9655, -2.7657) (-8.8753, -2.6594) (-8.8145, -2.5445) (-8.7829, -2.4207) knots 0 0 0 0 1 1 1 1
  spline S635 degree 3 poles (-8.7829, -2.4207) (-9.4149, -2.8072) (-10.0981, -2.9493) (-10.8325, -2.8469) knots 0 0 0 0 1 1 1 1
  spline S636 degree 3 poles (-10.8325, -2.8469) (-11.3953, -2.7169) (-11.7403, -2.3719) (-11.8674, -1.8119) knots 0 0 0 0 1 1 1 1
  spline S637 degree 3 poles (-11.8674, -1.8119) (-12.4436, -2.2658) (-13.0862, -2.5972) (-13.7952, -2.8063) knots 0 0 0 0 1 1 1 1
  spline S638 degree 3 poles (-13.7952, -2.8063) (-14.1315, -2.8653) (-14.4697, -2.8788) (-14.8099, -2.8469) knots 0 0 0 0 1 1 1 1
  spline S639 degree 3 poles (-14.8099, -2.8469) (-15.1554, -2.7719) (-15.4057, -2.5757) (-15.5607, -2.2584) knots 0 0 0 0 1 1 1 1
  spline S640 degree 3 poles (-15.5607, -2.2584) (-16.0968, -2.682) (-16.7056, -2.9255) (-17.3871, -2.9889) knots 0 0 0 0 1 1 1 1
  spline S641 degree 3 poles (-17.3871, -2.9889) (-18.5386, -2.9198) (-19.0932, -2.311) (-19.0511, -1.1626) knots 0 0 0 0 1 1 1 1
  spline S642 degree 3 poles (-19.0511, -1.1626) (-18.9093, -0.6489) (-18.6522, -0.2024) (-18.2799, 0.1768) knots 0 0 0 0 1 1 1 1
  spline S643 degree 3 poles (-18.2799, 0.1768) (-17.4808, 0.9859) (-16.5406, 1.5744) (-15.4592, 1.9423) knots 0 0 0 0 1 1 1 1
  spline S644 degree 3 poles (-15.4592, 1.9423) (-14.7726, 2.1501) (-14.0962, 2.1231) (-13.4299, 1.8611) knots 0 0 0 0 1 1 1 1
  spline S645 degree 3 poles (-13.4299, 1.8611) (-12.9721, 1.5926) (-12.7624, 1.1935) (-12.8009, 0.6638) knots 0 0 0 0 1 1 1 1
  spline S646 degree 3 poles (-12.8009, 0.6638) (-12.6002, 0.8751) (-12.3635, 0.936) (-12.0906, 0.8464) knots 0 0 0 0 1 1 1 1
  spline S647 degree 3 poles (-12.0906, 0.8464) (-11.82, 0.6164) (-11.82, 0.3865) (-12.0906, 0.1565) knots 0 0 0 0 1 1 1 1
  spline S648 degree 3 poles (-12.0906, 0.1565) (-12.9639, -0.3379) (-13.7688, -0.9264) (-14.5055, -1.609) knots 0 0 0 0 1 1 1 1
  spline S649 degree 3 poles (-14.5055, -1.609) (-14.5965, -1.7135) (-14.6709, -1.8285) (-14.7287, -1.954) knots 0 0 0 0 1 1 1 1
  spline S650 degree 3 poles (-14.7287, -1.954) (-14.7123, -1.9923) (-14.6852, -2.0194) (-14.6475, -2.0351) knots 0 0 0 0 1 1 1 1
  spline S651 degree 3 poles (-14.6475, -2.0351) (-14.2054, -2.0739) (-13.786, -1.9927) (-13.3894, -1.7916) knots 0 0 0 0 1 1 1 1
  spline S652 degree 3 poles (-13.3894, -1.7916) (-12.685, -1.4428) (-12.056, -0.9897) (-11.5021, -0.432) knots 0 0 0 0 1 1 1 1
  spline S653 degree 3 poles (-11.5021, -0.432) (-10.8474, 0.7367) (-9.9071, 1.5958) (-8.6814, 2.1452) knots 0 0 0 0 1 1 1 1
  spline S654 degree 3 poles (-8.6814, 2.1452) (-8.1756, 2.2085) (-7.9998, 1.9988) (-8.1538, 1.5161) knots 0 0 0 0 1 1 1 1
  spline S655 degree 3 poles (-8.1538, 1.5161) (-8.8418, 1.2026) (-9.4574, 0.7832) (-10.0004, 0.258) knots 0 0 0 0 1 1 1 1
  spline S656 degree 3 poles (-10.0004, 0.258) (-10.2034, 0.0009) (-10.4063, -0.2561) (-10.6092, -0.5132) knots 0 0 0 0 1 1 1 1
  spline S657 degree 3 poles (-10.6092, -0.5132) (-10.7757, -0.7957) (-10.911, -1.0934) (-11.0151, -1.4061) knots 0 0 0 0 1 1 1 1
  spline S658 degree 3 poles (-11.0151, -1.4061) (-11.1056, -1.7325) (-10.9907, -1.9422) (-10.6701, -2.0351) knots 0 0 0 0 1 1 1 1
  spline S659 degree 3 poles (-10.6701, -2.0351) (-10.3976, -2.064) (-10.127, -2.0505) (-9.8584, -1.9946) knots 0 0 0 0 1 1 1 1
  spline S660 degree 3 poles (-9.8584, -1.9946) (-9.1369, -1.7321) (-8.4808, -1.36) (-7.89, -0.8785) knots 0 0 0 0 1 1 1 1
  spline S661 degree 3 poles (-7.89, -0.8785) (-7.4165, -0.0126) (-6.943, 0.8532) (-6.4695, 1.719) knots 0 0 0 0 1 1 1 1
  spline S662 degree 3 poles (-6.4695, 1.719) (-6.199, 2.0742) (-5.854, 2.1756) (-5.4345, 2.0234) knots 0 0 0 0 1 1 1 1
  spline S663 degree 3 poles (-5.4345, 2.0234) (-5.1615, 1.795) (-5.0735, 1.5041) (-5.1707, 1.1508) knots 0 0 0 0 1 1 1 1
  spline S664 degree 3 poles (-5.1707, 1.1508) (-5.3537, 0.6163) (-5.6378, 0.1428) (-6.023, -0.2697) knots 0 0 0 0 1 1 1 1
  spline S665 degree 3 poles (-6.023, -0.2697) (-6.4045, -0.6782) (-6.8103, -1.057) (-7.2406, -1.4061) knots 0 0 0 0 1 1 1 1
  spline S666 degree 3 poles (-7.2406, -1.4061) (-7.3732, -1.6171) (-7.4815, -1.8336) (-7.5653, -2.0554) knots 0 0 0 0 1 1 1 1
  spline S667 degree 3 poles (-7.5653, -2.0554) (-6.7903, -1.6445) (-6.053, -1.1777) (-5.3534, -0.6552) knots 0 0 0 0 1 1 1 1
  spline S668 degree 3 poles (-5.3534, -0.6552) (-4.5999, 0.3711) (-3.6529, 1.1693) (-2.5124, 1.7393) knots 0 0 0 0 1 1 1 1
  spline S669 degree 3 poles (-2.5124, 1.7393) (-1.6846, 2.1155) (-0.8323, 2.1832) (0.0445, 1.9423) knots 0 0 0 0 1 1 1 1
  spline S670 degree 3 poles (0.0445, 1.9423) (0.2359, 1.86) (0.3982, 1.7382) (0.5316, 1.577) knots 0 0 0 0 1 1 1 1
  spline S671 degree 3 poles (0.5316, 1.577) (0.5586, 1.5499) (0.5857, 1.5499) (0.6127, 1.577) knots 0 0 0 0 1 1 1 1
  spline S672 degree 3 poles (0.6127, 1.577) (1.2648, 2.4997) (1.948, 3.3993) (2.6623, 4.2759) knots 0 0 0 0 1 1 1 1
  spline S673 degree 3 poles (2.6623, 4.2759) (2.9289, 4.5697) (3.2198, 4.8336) (3.5349, 5.0674) knots 0 0 0 0 1 1 1 1
  spline S674 degree 3 poles (3.5349, 5.0674) (4.2399, 5.1741) (4.5443, 4.8697) (4.4481, 4.1542) knots 0 0 0 0 1 1 1 1
  spline S675 degree 3 poles (4.4481, 4.1542) (4.3995, 3.9625) (4.3184, 3.7866) (4.2046, 3.6266) knots 0 0 0 0 1 1 1 1
  spline S676 degree 3 poles (4.2046, 3.6266) (3.7014, 3.0014) (3.1534, 2.4129) (2.5608, 1.8611) knots 0 0 0 0 1 1 1 1
  spline S677 degree 3 poles (2.5608, 1.8611) (1.8926, 1.2876) (1.2365, 0.6991) (0.5924, 0.0956) knots 0 0 0 0 1 1 1 1
  spline S678 degree 3 poles (0.5924, 0.0956) (0.1256, -0.5672) (-0.3006, -1.2571) (-0.686, -1.9743) knots 0 0 0 0 1 1 1 1
  spline S679 degree 3 poles (-0.686, -1.9743) (-0.4059, -2.0036) (-0.1353, -1.9562) (0.1257, -1.8322) knots 0 0 0 0 1 1 1 1
  spline S680 degree 3 poles (0.1257, -1.8322) (1.0853, -1.3734) (1.9173, -0.7443) (2.6217, 0.055) knots 0 0 0 0 1 1 1 1
  spline S681 degree 3 poles (2.6217, 0.055) (2.9798, 0.5006) (3.318, 0.9605) (3.6364, 1.4349) knots 0 0 0 0 1 1 1 1
  spline S682 degree 3 poles (3.6364, 1.4349) (3.6067, 1.6426) (3.5729, 1.8522) (3.5349, 2.064) knots 0 0 0 0 1 1 1 1
  spline S683 degree 3 poles (3.5349, 2.064) (3.5595, 2.4471) (3.7624, 2.6704) (4.1437, 2.7337) knots 0 0 0 0 1 1 1 1
  spline S684 degree 3 poles (4.1437, 2.7337) (4.4659, 2.7158) (4.6756, 2.5535) (4.7728, 2.2467) knots 0 0 0 0 1 1 1 1
  spline S685 degree 3 poles (4.7728, 2.2467) (4.784, 2.0854) (4.7908, 1.9298) (4.7931, 1.7799) knots 0 0 0 0 1 1 1 1
  spline S686 degree 3 poles (4.7931, 1.7799) (5.1055, 1.746) (5.4167, 1.7054) (5.7265, 1.6582) knots 0 0 0 0 1 1 1 1
  spline S687 degree 3 poles (5.7265, 1.6582) (6.0883, 1.5099) (6.2166, 1.2461) (6.1123, 0.8667) knots 0 0 0 0 1 1 1 1
  spline S688 degree 3 poles (6.1123, 0.8667) (6.0692, 0.7402) (6.0149, 0.6184) (5.9499, 0.5015) knots 0 0 0 0 1 1 1 1
  spline S689 degree 3 poles (5.9499, 0.5015) (5.6485, 0.0748) (5.3373, -0.3445) (5.0163, -0.7567) knots 0 0 0 0 1 1 1 1
  spline S690 degree 3 poles (5.0163, -0.7567) (4.7945, -1.0603) (4.6051, -1.385) (4.4481, -1.7308) knots 0 0 0 0 1 1 1 1
  spline S691 degree 3 poles (4.4481, -1.7308) (4.382, -1.9045) (4.3752, -2.0804) (4.4278, -2.2584) knots 0 0 0 0 1 1 1 1
  spline S692 degree 3 poles (4.4278, -2.2584) (4.4862, -2.2812) (4.5471, -2.2948) (4.6104, -2.299) knots 0 0 0 0 1 1 1 1
  spline S693 degree 3 poles (4.6104, -2.299) (5.4737, -2.0991) (6.2787, -1.7609) (7.0254, -1.2843) knots 0 0 0 0 1 1 1 1
  spline S694 degree 3 poles (7.0254, -1.2843) (7.1253, -0.7409) (7.3282, -0.2404) (7.6342, 0.2174) knots 0 0 0 0 1 1 1 1
  spline S695 degree 3 poles (7.6342, 0.2174) (7.4163, 0.5815) (7.5109, 0.825) (7.9183, 0.9479) knots 0 0 0 0 1 1 1 1
  spline S696 degree 3 poles (7.9183, 0.9479) (8.0068, 0.9441) (8.088, 0.917) (8.1619, 0.8667) knots 0 0 0 0 1 1 1 1
  spline S697 degree 3 poles (8.1619, 0.8667) (8.7353, 1.4174) (9.3847, 1.8571) (10.11, 2.1858) knots 0 0 0 0 1 1 1 1
  spline S698 degree 3 poles (10.11, 2.1858) (10.7857, 2.4482) (11.4489, 2.4212) (12.0987, 2.1046) knots 0 0 0 0 1 1 1 1
  spline S699 degree 3 poles (12.0987, 2.1046) (12.7566, 1.5763) (12.8446, 0.9608) (12.3625, 0.258) knots 0 0 0 0 1 1 1 1
  spline S700 degree 3 poles (12.3625, 0.258) (11.7805, -0.2999) (11.084, -0.584) (10.2723, -0.5943) knots 0 0 0 0 1 1 1 1
  spline S701 degree 3 poles (10.2723, -0.5943) (9.6221, -0.5586) (8.993, -0.4234) (8.3851, -0.1885) knots 0 0 0 0 1 1 1 1
  spline S702 degree 3 poles (8.3851, -0.1885) (8.0888, -0.5449) (7.9196, -0.9575) (7.8777, -1.4264) knots 0 0 0 0 1 1 1 1
  spline S703 degree 3 poles (7.8777, -1.4264) (7.8928, -1.6325) (7.9739, -1.8084) (8.1213, -1.954) knots 0 0 0 0 1 1 1 1
  spline S704 degree 3 poles (8.1213, -1.954) (8.2438, -1.9594) (8.3522, -2) (8.446, -2.0757) knots 0 0 0 0 1 1 1 1
  spline S705 degree 3 poles (8.446, -2.0757) (8.9366, -2.1144) (9.4237, -2.0873) (9.907, -1.9946) knots 0 0 0 0 1 1 1 1
  spline S706 degree 3 poles (9.907, -1.9946) (11.0333, -1.6547) (12.0479, -1.1136) (12.951, -0.3711) knots 0 0 0 0 1 1 1 1
  spline S707 degree 3 poles (12.951, -0.3711) (13.7099, 0.5701) (14.6434, 1.2872) (15.7514, 1.7799) knots 0 0 0 0 1 1 1 1
  spline S708 degree 3 poles (15.7514, 1.7799) (16.4036, 2.0727) (17.0798, 2.1539) (17.7807, 2.0234) knots 0 0 0 0 1 1 1 1
  spline S709 degree 3 poles (17.7807, 2.0234) (18.5116, 1.861) (18.8834, 1.4079) (18.8968, 0.6638) knots 0 0 0 0 1 1 1 1
  spline S710 degree 3 poles (18.8968, 0.6638) (19.0583, 0.836) (19.2543, 0.9104) (19.4853, 0.887) knots 0 0 0 0 1 1 1 1
  spline S711 degree 3 poles (19.4853, 0.887) (19.7568, 0.7823) (19.8445, 0.5861) (19.7491, 0.2985) knots 0 0 0 0 1 1 1 1
  spline S712 degree 3 poles (19.7491, 0.2985) (18.9755, -0.2043) (18.2247, -0.7387) (17.4966, -1.3046) knots 0 0 0 0 1 1 1 1
  spline S713 degree 3 poles (17.4966, -1.3046) (17.2742, -1.4862) (17.098, -1.7027) (16.969, -1.954) knots 0 0 0 0 1 1 1 1
  spline S714 degree 3 poles (16.969, -1.954) (16.9856, -1.9923) (17.0124, -2.0194) (17.0501, -2.0351) knots 0 0 0 0 1 1 1 1
  spline S715 degree 3 poles (17.0501, -2.0351) (17.4162, -2.0756) (17.7681, -2.0214) (18.1054, -1.8728) knots 0 0 0 0 1 1 1 1
  spline S716 degree 3 poles (18.1054, -1.8728) (19.0867, -1.4199) (19.9187, -0.7772) (20.6014, 0.055) knots 0 0 0 0 1 1 1 1
  spline S717 degree 3 poles (20.6014, 0.055) (20.9322, 0.4461) (21.2232, 0.8655) (21.474, 1.3132) knots 0 0 0 0 1 1 1 1
  spline S718 degree 3 poles (21.474, 1.3132) (21.2869, 1.7955) (21.4492, 2.0187) (21.961, 1.9828) knots 0 0 0 0 1 1 1 1
  spline S719 degree 3 poles (21.961, 1.9828) (22.2788, 1.7875) (22.4006, 1.5102) (22.3263, 1.1508) knots 0 0 0 0 1 1 1 1
  spline S720 degree 3 poles (22.3263, 1.1508) (22.9895, 1.6347) (23.7269, 1.9323) (24.5382, 2.0437) knots 0 0 0 0 1 1 1 1
  spline S721 degree 3 poles (24.5382, 2.0437) (25.1437, 2.0526) (25.5159, 1.7685) (25.6543, 1.1914) knots 0 0 0 0 1 1 1 1
  spline S722 degree 3 poles (10.7999, 0.8667) (10.5828, 0.7924) (10.3665, 0.7045) (10.1506, 0.6029) knots 0 0 0 0 1 1 1 1
  spline S723 degree 3 poles (10.1506, 0.6029) (10.5418, 0.5621) (10.9071, 0.6432) (11.2464, 0.8464) knots 0 0 0 0 1 1 1 1
  spline S724 degree 3 poles (11.2464, 0.8464) (11.0982, 0.8667) (10.9493, 0.8734) (10.7999, 0.8667) knots 0 0 0 0 1 1 1 1
  spline S725 degree 3 poles (-1.1325, 0.6232) (-2.2555, 0.3285) (-3.2092, -0.2533) (-3.9938, -1.122) knots 0 0 0 0 1 1 1 1
  spline S726 degree 3 poles (-3.9938, -1.122) (-4.1157, -1.269) (-4.1969, -1.4313) (-4.2373, -1.609) knots 0 0 0 0 1 1 1 1
  spline S727 degree 3 poles (-4.2373, -1.609) (-4.1708, -1.7027) (-4.0829, -1.7636) (-3.9735, -1.7916) knots 0 0 0 0 1 1 1 1
  spline S728 degree 3 poles (-3.9735, -1.7916) (-3.69, -1.836) (-3.4194, -1.7954) (-3.1617, -1.6699) knots 0 0 0 0 1 1 1 1
  spline S729 degree 3 poles (-3.1617, -1.6699) (-2.1944, -1.1222) (-1.3624, -0.4119) (-0.6657, 0.4609) knots 0 0 0 0 1 1 1 1
  spline S730 degree 3 poles (-0.6657, 0.4609) (-0.6205, 0.512) (-0.6138, 0.5594) (-0.6454, 0.6029) knots 0 0 0 0 1 1 1 1
  spline S731 degree 3 poles (-0.6454, 0.6029) (-0.8072, 0.6232) (-0.9695, 0.63) (-1.1325, 0.6232) knots 0 0 0 0 1 1 1 1
  spline S732 degree 3 poles (-14.8099, 0.5826) (-16.001, 0.2541) (-16.9818, -0.3953) (-17.7523, -1.3655) knots 0 0 0 0 1 1 1 1
  spline S733 degree 3 poles (-17.7523, -1.3655) (-17.916, -1.5781) (-17.8686, -1.7202) (-17.6103, -1.7916) knots 0 0 0 0 1 1 1 1
  spline S734 degree 3 poles (-17.6103, -1.7916) (-17.4615, -1.8187) (-17.3127, -1.8187) (-17.1638, -1.7916) knots 0 0 0 0 1 1 1 1
  spline S735 degree 3 poles (-17.1638, -1.7916) (-16.7697, -1.6554) (-16.4044, -1.4661) (-16.068, -1.2234) knots 0 0 0 0 1 1 1 1
  spline S736 degree 3 poles (-16.068, -1.2234) (-15.3561, -0.7146) (-14.7067, -0.1328) (-14.1199, 0.5218) knots 0 0 0 0 1 1 1 1
  spline S737 degree 3 poles (-14.1199, 0.5218) (-14.3424, 0.5806) (-14.5724, 0.6009) (-14.8099, 0.5826) knots 0 0 0 0 1 1 1 1
  spline S738 degree 3 poles (16.8878, 0.5826) (16.6881, 0.5291) (16.4852, 0.4682) (16.279, 0.4) knots 0 0 0 0 1 1 1 1
  spline S739 degree 3 poles (16.279, 0.4) (15.2944, -0.0031) (14.4896, -0.6321) (13.8642, -1.4872) knots 0 0 0 0 1 1 1 1
  spline S740 degree 3 poles (13.8642, -1.4872) (13.8341, -1.566) (13.8406, -1.6404) (13.8844, -1.7105) knots 0 0 0 0 1 1 1 1
  spline S741 degree 3 poles (13.8844, -1.7105) (14.1799, -1.8416) (14.4774, -1.8416) (14.7773, -1.7105) knots 0 0 0 0 1 1 1 1
  spline S742 degree 3 poles (14.7773, -1.7105) (15.1357, -1.5382) (15.4738, -1.3352) (15.792, -1.1017) knots 0 0 0 0 1 1 1 1
  spline S743 degree 3 poles (15.792, -1.1017) (16.4174, -0.6385) (16.9925, -0.1177) (17.5169, 0.4609) knots 0 0 0 0 1 1 1 1
  spline S744 degree 3 poles (17.5169, 0.4609) (17.5364, 0.4994) (17.5433, 0.5399) (17.5372, 0.5826) knots 0 0 0 0 1 1 1 1
  spline S745 degree 3 poles (17.5372, 0.5826) (17.3208, 0.5826) (17.1041, 0.5826) (16.8878, 0.5826) knots 0 0 0 0 1 1 1 1
  spline S746 degree 3 poles (3.332, 2.0843) (3.359, 1.8814) (3.3861, 1.6785) (3.4132, 1.4755) knots 0 0 0 0 1 1 1 1
  spline S747 degree 3 poles (3.4132, 1.4755) (3.4192, 1.4328) (3.4125, 1.3922) (3.3929, 1.3538) knots 0 0 0 0 1 1 1 1
  spline S748 degree 3 poles (3.3929, 1.3538) (2.6691, 0.2512) (1.7559, -0.662) (0.6533, -1.3858) knots 0 0 0 0 1 1 1 1
  spline S749 degree 3 poles (0.6533, -1.3858) (0.3788, -1.5437) (0.0947, -1.6654) (-0.199, -1.751) knots 0 0 0 0 1 1 1 1
  spline S750 degree 3 poles (-0.199, -1.751) (0.1037, -1.2469) (0.4217, -0.7531) (0.7548, -0.2697) knots 0 0 0 0 1 1 1 1
  spline S751 degree 3 poles (0.7548, -0.2697) (1.6461, 0.4796) (2.5052, 1.2643) (3.332, 2.0843) knots 0 0 0 0 1 1 1 1
  spline S752 degree 3 poles (3.1696, 1.6785) (2.4119, 0.9411) (1.634, 0.2241) (0.836, -0.4726) knots 0 0 0 0 1 1 1 1
  spline S753 degree 3 poles (0.836, -0.4726) (0.6736, -0.7161) (0.5113, -0.9596) (0.3489, -1.2031) knots 0 0 0 0 1 1 1 1
  spline S754 degree 3 poles (0.3489, -1.2031) (0.3091, -1.2542) (0.2956, -1.3083) (0.3083, -1.3655) knots 0 0 0 0 1 1 1 1
  spline S755 degree 3 poles (0.3083, -1.3655) (1.4523, -0.6846) (2.3993, 0.2083) (3.1493, 1.3132) knots 0 0 0 0 1 1 1 1
  spline S756 degree 3 poles (3.1493, 1.3132) (3.2168, 1.4374) (3.2236, 1.5591) (3.1696, 1.6785) knots 0 0 0 0 1 1 1 1
  spline S757 degree 3 poles (3.332, 2.0843) (3.3344, 2.1063) (3.3479, 2.1199) (3.3726, 2.1249) knots 0 0 0 0 1 1 1 1
  spline S758 degree 3 poles (3.3726, 2.1249) (3.4129, 1.9101) (3.4265, 1.6937) (3.4132, 1.4755) knots 0 0 0 0 1 1 1 1
  spline S759 degree 3 poles (3.4132, 1.4755) (3.3861, 1.6785) (3.359, 1.8814) (3.332, 2.0843) knots 0 0 0 0 1 1 1 1
  spline S760 degree 3 poles (10.7999, 1.5567) (11.1835, 1.6282) (11.515, 1.5335) (11.7943, 1.2726) knots 0 0 0 0 1 1 1 1
  spline S761 degree 3 poles (11.7943, 1.2726) (11.8694, 1.1523) (11.8694, 1.0306) (11.7943, 0.9073) knots 0 0 0 0 1 1 1 1
  spline S762 degree 3 poles (11.7943, 0.9073) (11.5597, 0.6332) (11.2691, 0.437) (10.9217, 0.3188) knots 0 0 0 0 1 1 1 1
  spline S763 degree 3 poles (10.9217, 0.3188) (10.2553, 0.1542) (9.6059, 0.2083) (8.9736, 0.4812) knots 0 0 0 0 1 1 1 1
  spline S764 degree 3 poles (8.9736, 0.4812) (9.4991, 0.9873) (10.1079, 1.3458) (10.7999, 1.5567) knots 0 0 0 0 1 1 1 1
  spline S765 degree 3 poles (10.7999, 0.8667) (10.5828, 0.7924) (10.3665, 0.7045) (10.1506, 0.6029) knots 0 0 0 0 1 1 1 1
  spline S766 degree 3 poles (10.1506, 0.6029) (10.5418, 0.5621) (10.9071, 0.6432) (11.2464, 0.8464) knots 0 0 0 0 1 1 1 1
  spline S767 degree 3 poles (11.2464, 0.8464) (11.0982, 0.8667) (10.9493, 0.8734) (10.7999, 0.8667) knots 0 0 0 0 1 1 1 1
  spline S768 degree 3 poles (-1.376, 1.2726) (-1.0915, 1.2793) (-0.8074, 1.2726) (-0.5237, 1.2523) knots 0 0 0 0 1 1 1 1
  spline S769 degree 3 poles (-0.5237, 1.2523) (-0.3633, 1.2305) (-0.2213, 1.1697) (-0.0975, 1.0697) knots 0 0 0 0 1 1 1 1
  spline S770 degree 3 poles (-0.0975, 1.0697) (-0.0814, 0.8499) (-0.1356, 0.647) (-0.2599, 0.4609) knots 0 0 0 0 1 1 1 1
  spline S771 degree 3 poles (-0.2599, 0.4609) (-0.9077, -0.4441) (-1.6991, -1.1949) (-2.6341, -1.7916) knots 0 0 0 0 1 1 1 1
  spline S772 degree 3 poles (-2.6341, -1.7916) (-3.0819, -2.0795) (-3.5689, -2.1877) (-4.0952, -2.1163) knots 0 0 0 0 1 1 1 1